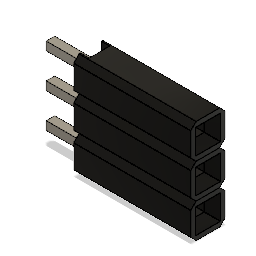
pinsStraightFemale (Autodesk Fusion 360 design; units mm, degrees)
Autodesk Fusion 360 part; units mm, degrees
sketch "Sketch1" plane through (0, 0, 0) normal (0, 1, 0) x (1, 0, 0) in component "Pin"
  line L0 (0, 0) -> (5.08, 0)
  line L1 (5.08, 0) -> (5.08, -0.635)
  line L2 (5.08, -0.635) -> (0, -0.635)
  line L3 (0, -0.635) -> (0, 0)
  dimension "d2" = 0.635
  dimension "d3" = 5.08
  measures "d3" distance of L0.start
extrude "Extrude1" add sketch "Sketch1" along normal blind 0.635 makes body 1 in component "Pin"
chamfer "Chamfer1" distance 0.1905 angle 45 4 edges at (0, 0.3175, 0.635) (0, 0.635, 0.3175) (0, 0.3175, 0) (0, 0, 0.3175) on bodies 1 in component "Pin"
sketch "Sketch1 (2)" plane through (0, 0, 0) normal (0, 1, 0) x (1, 0, 0) in component "Plastic"
  line L0 (0, -0.3175) -> (3.81, -0.3175)
  line L1 (3.81, -1.0795) -> (3.81, 0.4445)
  line L2 (3.81, 0.4445) -> (3.8102, 0.9525) construction
  line L3 (3.81, -1.0795) -> (3.81, -1.5875) construction
  line L4 (3.81, 0.4445) -> (3.175, 0.4445)
  line L5 (3.81, -1.0795) -> (3.175, -1.0795)
  line L6 (3.175, -1.0795) -> (3.175, -1.5875)
  line L7 (3.175, 0.4445) -> (3.175, 0.9525)
  line L8 (3.175, 0.9525) -> (11.811, 0.9525)
  line L9 (11.811, 0.9525) -> (11.811, -1.5875)
  line L10 (3.175, -1.5875) -> (11.811, -1.5875)
  line L11 (0, -0.1905) -> (0, -0.4445)
  dimension "d7" = 3.81
  dimension "d8" = 1.524
  dimension "d9" = 0.508
  dimension "d11" = 0.635
  dimension "d12" = 8.636
  measures "d7" distance of origin
extrude "Extrude1'" add sketch "Sketch1 (2)" along normal mid plane 2.54 from surface at 0.3175 separate body makes body 2 in component "Plastic"
chamfer "Chamfer1'" distance 0.4 angle 45 4 edges at (7.493, 1.5875, -0.9525) (7.493, -0.9525, -0.9525) (7.493, 1.5875, 1.5875) (7.493, -0.9525, 1.5875) on bodies 2 in component "Plastic"
sketch "Sketch1 (3)" plane through (0, 0, 0) normal (0, 0, 1) x (1, 0, 0)
  line L0 (0, 0.1905) -> (0, 0.4445)
  line L1 (0, 0.3175) -> (0, 14)
other "PathPattern1" in component "Header"
sketch "Sketch1 (1)" plane through (11.811, 0, 0) normal (1, 0, 0) x (0, 0, -1) in component "Plastic"
  line L0 (-1.5875, -0.5525) -> (-1.1875, -0.9525)
  line L1 (-1.1875, -0.9525) -> (0.5525, -0.9525)
  line L2 (0.5525, -0.9525) -> (0.9525, -0.5525)
  line L3 (0.9525, -0.5525) -> (0.9525, 1.1875)
  line L4 (0.9525, 1.1875) -> (0.5525, 1.5875)
  line L5 (0.5525, 1.5875) -> (-1.1875, 1.5875)
  line L6 (-1.1875, 1.5875) -> (-1.5875, 1.1875)
  line L7 (-1.5875, 1.1875) -> (-1.5875, -0.5525)
  line L8 (0.9525, 0.3175) -> (-0.3175, 0.3175) construction
  line L9 (-0.3175, 1.5875) -> (-0.3175, 0.3175) construction
  line L10 (-0.3175, 0.635) -> (0, 0.635)
  line L11 (0, 0.3175) -> (0, 0)
  line L12 (0, 0) -> (-0.635, 0)
  line L13 (-0.635, 0) -> (-0.635, 0.635)
  line L14 (0, 0.635) -> (0, 0.3175)
  line L15 (-0.635, 0.635) -> (-0.3175, 0.635)
  dimension "d24" = 0.635
  dimension "d25" = 0.635
  measures "d25" distance of L11.end
extrude "Extrude1''" cut sketch "Sketch1 (1)" against normal blind 5.5 contours L10 L11 L12 L13 L14 L15 bodies 2 in component "Plastic"
chamfer "Chamfer1''" distance 0.6 angle 45 4 edges at (11.811, 0, 0.3175) (11.811, 0.3175, 0) (11.811, 0.635, 0.3175) (11.811, 0.3175, 0.635) on bodies 2 in component "Plastic"
component "Header" placed x (1, 0, 0) y (0, 1, 0) z (0, 0, 1) at (0, 0, 0)
component "Header" placed x (1, 0, 0) y (0, 1, 0) z (0, 0, 1) at (0, 2.54, 0)
component "Header" placed x (1, 0, 0) y (0, 1, 0) z (0, 0, 1) at (0, 5.08, 0)
component "Pin" placed x (1, 0, 0) y (0, 1, 0) z (0, 0, 1) at (0, 0, 0) in component "Header"
component "Plastic" placed x (1, 0, 0) y (0, 1, 0) z (0, 0, 1) at (0, 0, 0) in component "Header"
equation "pinCount = 3"
equation "d12 = plasticHeight"
equation "d13 = 0.025 in / 2"
equation "d19 = pinCount"
equation "d21 = pinCount"
equation "plasticHeight = 0.34 in"
